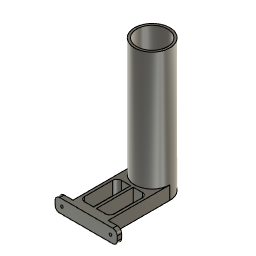
toilet-roll-holder v3 (Autodesk Fusion 360 design; units mm, degrees)
Autodesk Fusion 360 part; units mm, degrees
sketch "Sketch1" plane through (0, 0, 0) normal (0, 0, 1) x (1, 0, 0)
  circle A0 centre (0, 0) radius 20
  dimension "d1" = 40
  constraint coincident A0.centre origin
  measures "d1" diameter of A0
extrude "Extrude1" add sketch "Sketch1" along normal blind 150 makes body 1
sketch "Sketch2" plane through (0, 0, 0) normal (0, 1, 0) x (1, 0, 0)
  line L0 (-20, 0) -> (20, 0) construction
  line L1 (-20, -150) -> (20, -150) construction
  line L2 (0, -150) -> (0, 0) construction
  line L3 (-20, -150) -> (-20, 0) construction
  line L4 (-20, 0) -> (-35.25, 0)
  line L5 (-35.25, 0) -> (-35.25, -15.25)
  line L6 (-35.25, -15.25) -> (-20, -15.25)
  line L7 (-27.625, -15.25) -> (-27.625, 0) construction
  circle A0 centre (-27.625, -7.625) radius 2.625
  circle A1 centre (-27.625, -7.625) radius 1.5
  line L8 (-20, -15.25) -> (0, -15.25)
  line L9 (-20, 0) -> (0, 0)
  line L10 (20, -15.25) -> (0, -15.25)
  line L11 (35.25, -15.25) -> (20, -15.25)
  line L12 (35.25, 0) -> (35.25, -15.25)
  line L13 (20, 0) -> (35.25, 0)
  line L14 (20, 0) -> (0, 0)
  circle A2 centre (27.625, -7.625) radius 2.625
  circle A3 centre (27.625, -7.625) radius 1.5
  line L15 (20, -15.25) -> (20, 0)
  line L16 (-20, -15.25) -> (-20, 0)
  line L17 (20, -15.25) -> (20, 0)
  line L18 (-20, -15.25) -> (-20, 0)
  point P0 (-27.625, -7.625)
  dimension "d5" = 5.25
  dimension "d6" = 3
  dimension "d7" = 5
  dimension "d8" = 5
  dimension "d13" = 5
  constraint midpoint L1 L2.start
  constraint coincident L2.end L9.end
  constraint coincident L1.start L3.start
  constraint coincident L0.start L3.end
  constraint perpendicular L3 L4
  constraint perpendicular L0 L5
  constraint coincident L3 L6.end
  constraint perpendicular L3 L6
  constraint midpoint L6 L7.start
  constraint midpoint L4 L7.end
  constraint midpoint L7 P0
  constraint coincident P0 A0.centre
  constraint coincident L2 L8.end
  constraint perpendicular L2 L8
  constraint symmetric L2 L0.start L0.end
  constraint symmetric L2 L4.end L12.start
  constraint symmetric L2 L5.end L11.start
  constraint symmetric L2 L6.end L10.start
  constraint symmetric L2 A0 A2
  constraint symmetric L2 A1 A3
  constraint symmetric L2 L8.end L10.end
  constraint symmetric L2 L9.end L14.end
  constraint symmetric L2 L10.start L6.end
  constraint symmetric L2 L0.end L0.start
  constraint coincident L11 L10.start
  constraint coincident L13 L0.end
  constraint perpendicular L13 L17
  measures "d5" diameter of A0
  measures "d6" diameter of A1
  measures "d7" distance of L6 A0
  measures "d8" distance of L5 A0
  measures "d13" distance of A2 L17
ref_plane "WorkPlane1" through (0, -20, 103.4458) normal (0, -1, 0) x (-1, 0, 0)
extrude "Extrude2" add sketch "Sketch2" against normal blind 55 from surface at -20 separate body contours L4 L5 L6 L16 L18 | L8 L9 L10 L14 L15 L16 L17 L18 | L11 L12 L13 L15 L17 | A0 | A2 makes body 2
extrude "Extrude3" add sketch "Sketch2" along normal blind 20 from surface at -20 contours L8 L9 L10 L14 L15 L16 L17 L18 bodies 1 2
move_face "OffsetFaces1" offset -50 2 faces at (27.6624, -20, 13.2069) (-27.5876, -20, 13.2069) on bodies 1
extrude "Extrude4" cut sketch "Sketch2" against normal blind 2.5 from surface at -70 contours A0 | A2 bodies 1
fillet "Fillet1" radius 5 4 edges at (35.25, -72.5, 15.25) (35.25, -72.5, 0) (-35.25, -72.5, 15.25) (-35.25, -72.5, 0) on bodies 1
sketch "Sketch3" plane through (0, 0, 15.25) normal (0, 0, 1) x (-1, 0, 0)
  line L0 (30.25, 70) -> (30.25, 75)
  line L1 (30.25, 75) -> (-30.25, 75)
  line L2 (-30.25, 75) -> (-30.25, 70)
  line L3 (-30.25, 70) -> (-20, 70)
  line L4 (-20, 70) -> (-20, 0)
  arc A0 (20, 0) -> (-20, 0) centre (0, 0) ccw
  line L5 (20, 0) -> (20, 70)
  line L6 (20, 70) -> (30.25, 70)
  line L7 (-30.25, 75) -> (30.25, 75)
  line L8 (20, 70) -> (20, 0)
  line L9 (-20, 70) -> (-20, 0)
  circle A1 centre (0, 0) radius 20
  line L10 (0, 75) -> (0, 20) construction
  line L11 (17, 23) -> (-17, 23)
  line L12 (-17, 23) -> (-17, 65)
  line L13 (-17, 65) -> (17, 65)
  line L14 (17, 65) -> (17, 23)
  circle A2 centre (0, 0) radius 17.5
  line L15 (-1.5, 65) -> (-1.5, 23)
  line L16 (1.5, 65) -> (1.5, 23)
  dimension "d23" = 3
  dimension "d24" = 3
  dimension "d25" = 5
  dimension "d26" = 3
  dimension "d31" = -2.5
  dimension "d41" = 1.5
  constraint midpoint L7 L10.start
  constraint midpoint A0 L10.end
  constraint horizontal L11
  constraint vertical L12
  constraint horizontal L13
  constraint vertical L14
  constraint coincident L13 L15.start
  constraint coincident L11 L15.end
  constraint perpendicular L11 L15
  constraint symmetric L10 L15.start L16.start
  constraint symmetric L10 L15.end L16.end
  measures "d23" distance of L8 L14
  measures "d24" distance of L9 L12
  measures "d25" distance of L3 L13
  measures "d26" distance of A1 L11
  measures "d41" distance of L10 L15
extrude "Extrude5" cut sketch "Sketch3" against normal up to surface (15.25 mm away) contours L11 L13 L14 L16 | L11 L12 L13 L15 bodies 1
fillet "Fillet2" radius 5 4 edges at (-17, -65, 7.625) (-17, -23, 7.625) (17, -23, 7.625) (17, -65, 7.625) on bodies 1
extrude "Extrude6" cut sketch "Sketch3" against normal up to surface (150 mm away) from surface at 134.75 contours A2 bodies 1
sketch "Sketch4" plane through (20, 0, 0) normal (1, 0, 0) x (0, 1, 0)
  line L0 (-70, 15.25) -> (-70, 0)
  line L1 (-70, 0) -> (0, 0)
  line L2 (0, 0) -> (0, 15.25)
  line L3 (0, 15.25) -> (-70, 15.25)
  line L4 (-66, 4) -> (-4, 4)
  line L5 (-4, 4) -> (-4, 11.25)
  line L6 (-4, 11.25) -> (-66, 11.25)
  line L7 (-66, 11.25) -> (-66, 4)
  line L8 (0, 15.25) -> (-20, 15.25)
  line L9 (-20, 15.25) -> (-20, 0) construction
  line L10 (-24, 15.25) -> (-24, 0)
  dimension "d35" = -4
  dimension "d36" = 4
  constraint coincident L8.end L9.start
  constraint coincident L1 L9.end
  constraint perpendicular L1 L9
  constraint coincident L3 L10.start
  constraint coincident L1 L10.end
  constraint perpendicular L1 L10
  measures "d36" distance of L9 L10
named bodies: "toilet-roll-holder"
